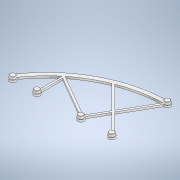
# Autodesk Inventor part: W-Support
Saved by Autodesk Inventor 2022.1 (Build 261234000, 234)
## iProperties
Company: El Camino College
Created: 2023-04-19
Part Number: W-Support
Material: ABS Plastic
Document SubType Name: Modeling
Designer: Edgar Tejada
Density: 1.06 g/cm^3
Appearance: Smooth - White
Mass: 8.73067 g
Surface Area: 83.9142 cm^2
Volume: 8.23648 cm^3
Description: Right Side of the Road with Middle Plugs
Author: Edgar Tejada
Title: West Side Road
Autodesk Inventor part; units mm, degrees
ref_plane "YZ Plane" through (0, 0, 0) normal (1, 0, 0) x (0, 1, 0)
ref_plane "XZ Plane" through (0, 0, 0) normal (0, 1, 0) x (-1, 0, 0)
ref_plane "XY Plane" through (0, 0, 0) normal (0, 0, 1) x (1, 0, 0)
sketch "Sketch1" plane through (0, 0, 0) normal (0, 1, 0) x (-1, 0, 0)
  arc A0 (-152, 0) -> (152, 0) centre (0, 100) ccw
  line L0 (0, -81.945) -> (-47.311, 0)
  line L1 (-47.311, 0) -> (47.311, 0) construction
  line L2 (47.311, 0) -> (0, -81.945)
  line L3 (0, 0) -> (68.5411, -68.5411)
  line L4 (0, 0) -> (-68.5411, -68.5411)
  line L5 (47.311, 0) -> (116.3651, -39.8684)
  line L6 (-47.311, 0) -> (-116.3651, -39.8684)
  line L7 (114.7776, -42.618) -> (48.4731, -4.3371)
  line L8 (48.4731, -4.3371) -> (0, -88.295)
  line L9 (0, -88.295) -> (-48.4731, -4.3371)
  line L10 (-48.4731, -4.3371) -> (-114.4332, -42.4192)
  line L11 (-66.0999, -70.5901) -> (0, -4.4901)
  line L12 (0, -4.4901) -> (66.2961, -70.7862)
  line L13 (116.3651, -39.8684) -> (114.7776, -42.618)
  line L14 (68.5411, -68.5411) -> (66.2961, -70.7862)
  line L15 (-66.0999, -70.5901) -> (-67.8825, -68.8075)
  line L16 (-114.4332, -42.4192) -> (-115.4867, -40.5945)
  arc A1 (-157.2837, -3.5223) -> (157.2837, -3.5223) centre (0, 100) ccw
  line L17 (157.2837, -3.5223) -> (152, 0)
  line L18 (-152, 0) -> (-157.2837, -3.5223)
  line L19 (116.3651, -39.8684) -> (113.3651, -39.8684)
  line L20 (113.3651, -39.8684) -> (113.3651, 0)
  line L21 (113.3651, 0) -> (116.3651, 0)
  line L22 (116.3651, 0) -> (116.3651, -39.8684)
  line L23 (0, 0) -> (0, -27.315) construction
  line L24 (-116.3651, -39.8684) -> (-113.3651, -39.8684)
  line L25 (-113.3651, -39.8684) -> (-113.3651, 0)
  line L26 (-113.3651, 0) -> (-116.3651, 0)
  line L27 (-116.3651, 0) -> (-116.3651, -39.8684)
  point P0 (-3.6878, -81.9077)
  point P1 (-65.3239, -69.814)
  point P2 (-30.6747, -35.1649)
  point P3 (29.994, -29.994)
  point P4 (-29.994, -29.994)
  point P5 (32.3182, -32.3182)
  point P6 (113.7344, -42.0158)
  point P7 (30.6747, -35.1649)
  point P8 (65.3239, -69.814)
  point P9 (3.6878, -81.9077)
  point P10 (-28.3505, -32.8406)
  point P11 (28.3505, -32.8406)
  point P12 (-32.3182, -32.3182)
  point P13 (-113.7344, -42.0158)
  point P14 (-113.3651, -38.1363)
  point P15 (113.3651, -38.1363)
  point P16 (0, 0)
  dimension "d0" = 152
  dimension "d1" = 152
  dimension "d2" = 100
  dimension "d3" = 0
  dimension "d4" = 45
  dimension "d8" = 3.175
  dimension "d9" = 3.175
  dimension "d10" = 6.35
  dimension "d11" = 6.35
  dimension "d12" = 3.5223
  dimension "d13" = 3.5223
  dimension "d29" = 3
  dimension "d30" = 157.2837
  constraints: 56 end point, 8 perpendicular, 3 horizontal alignment, 3 symmetric about line, 2 horizontal, 2 parallel, 2 point on circle, 1 centre point, 1 collinear, 1 midpoint, 22 other
  measures "d0" distance of L17.end L3.start
  measures "d1" distance of L18.start L3.start
  measures "d2" distance of A1.centre L3.start
  measures "d3" vertical distance of L3.start L0.end
  measures "d4" angle of L1 L4
  measures "d8" distance between parallel lines of L5 L7
  measures "d9" distance between parallel lines of L4 L11
  measures "d10" distance of L8.end L0.start
  measures "d12" vertical distance of L18.start L18.end
  measures "d13" vertical distance of L17.start L17.end
  measures "d29" distance of L5.end L19.end
  measures "d30" horizontal distance of point (0, 0) L17.start
extrude "Extrusion1" add sketch "Sketch1" along normal mid plane 3 contours A0 L16 L10 L15 L11 L9 A1 L18 | L24 L25 L6 L0 L4 L9 L10 A0 | L27 L26 L25 L6 | L6 L25 L24 | A0 L10 L16 | L9 A0 L8 | L8 A0 L12 L14 L7 L13 L17 A1 | A0 L2 L12 L8 | L9 L11 L0 A0 | L4 L9 L11 A0 | L4 L3 L2 L12 L11 L0 | L0 L11 L9 L4 | L12 L8 L3 A0 | A0 L14 L12 | L12 L2 L3 L8 | L11 L15 A0 | L3 L2 L5 L20 L19 A0 L7 L8 | L13 L7 A0 | L19 L20 L5 | L5 L20 L21 L22
sketch "Sketch2" plane through (0, 1.5, 0) normal (0, 1, 0) x (1, 0, 0)
  line L0 (0, 0) -> (29.994, 29.994) projected
  line L1 (0, 0) -> (200, 0)
  line L2 (200, 0) -> (200, 200)
  line L3 (200, 200) -> (0, 200)
  line L4 (0, 200) -> (0, 0)
  dimension "d16" = 200
  dimension "d17" = 200
  constraints: 8 end point, 2 parallel, 1 horizontal, 1 perpendicular
  measures "d16" distance of L2.end L3.end
  measures "d17" distance of L1.end L2.end
extrude "Extrusion2" cut sketch "Sketch2" along normal through all both and the other way through all
sketch "Sketch3" plane through (0, 1.5, 0) normal (0, 1, 0) x (1, 0, 0)
  line L0 (-29.994, 29.994) -> (0, 0) projected
  circle A0 centre (0, 0) radius 5
  line L1 (-157.2837, 3.5223) -> (-152, 0) projected
  line L2 (-47.311, 0) -> (-29.994, 29.994) projected
  circle A1 centre (-47.311, 0) radius 5
  line L3 (0, 81.945) -> (0, 88.295) projected
  circle A2 centre (0, 85.12) radius 5
  circle A3 centre (-152, 0) radius 5
  line L4 (-116.3651, 0) -> (-113.3651, 0) projected
  circle A4 centre (-114.8651, 0) radius 5
  dimension "d20" = 10
  constraints: 5 centre point, 4 equal radius, 2 coincident, 2 midpoint
  measures "d20" diameter of A2
extrude "Circular_Mounts" add sketch "Sketch3" against normal blind 3
sketch "Sketch4" plane through (0, 1.5, 0) normal (0, 1, 0) x (1, 0, 0)
  arc A0 (-51.6411, 2.5) -> (-44.811, 4.3301) centre (-47.311, 0) ccw projected
  circle A1 centre (-47.311, 0) radius 4.05
  circle A2 centre (0, 0) radius 4.05
  arc A3 (-156.1603, 2.7735) -> (-149.1948, 4.1389) centre (-152, 0) ccw projected
  circle A4 centre (-152, 0) radius 4.05
  arc A5 (-0.9958, 80.2202) -> (-3.8953, 88.2548) centre (0, 85.12) ccw projected
  circle A6 centre (0, 85.12) radius 4.05
  arc A7 (-116.3651, 4.7697) -> (-113.3651, 4.7697) centre (-114.8651, 0) ccw projected
  circle A8 centre (-114.8651, 0) radius 4.05
  dimension "d23" = 8.1
  constraints: 5 centre point, 5 coincident, 4 equal radius
  measures "d23" diameter of A6
extrude "Inserts" add sketch "Sketch4" along normal blind 4
fillet "Fillet2" radius 0.5 5 edges at (-156.05, 5.5, 0) (-51.361, 5.5, 0) (-4.05, 5.5, 0) (-4.05, 5.5, -85.12) (-118.9151, 5.5, 0)
fillet "Fillet3" radius 2 2 edges at (-156.1603, 0, -2.7735) (-157.2837, 0, -3.5223)
equation "\"d1\" = d0"
body "Solid1"
